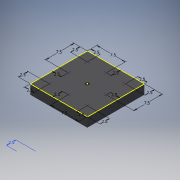
# Autodesk Inventor part: ClampCover
Saved by Autodesk Inventor 2016 (Build 200138000, 138)
## iProperties
Created: 2016-04-15
Part Number: ClampCover
Material: Generic
Document SubType Name: Modeling
Designer: Andres
Density: 1 g/cm^3
Appearance: Gray
Author: Andres
Autodesk Inventor part; units mm, degrees
ref_plane "YZ Plane" through (0, 0, 0) normal (1, 0, 0) x (0, 1, 0)
ref_plane "XZ Plane" through (0, 0, 0) normal (0, 1, 0) x (-1, 0, 0)
ref_plane "XY Plane" through (0, 0, 0) normal (0, 0, 1) x (1, 0, 0)
sketch "Sketch1" plane through (0, 0, 0) normal (0, 0, 1) x (1, 0, 0)
  line L0 (-7.5, 7.5) -> (7.5, 7.5)
  line L1 (7.5, 7.5) -> (7.5, -7.5)
  line L2 (7.5, -7.5) -> (-7.5, -7.5)
  line L3 (-7.5, -7.5) -> (-7.5, 7.5)
  point P0 (0, 0)
  point P1 (-7.5, 0)
  point P2 (0, 7.5)
  dimension "d0" = 15
  dimension "d1" = 15
  constraints: 8 end point, 2 midpoint, 2 parallel, 1 horizontal, 1 horizontal alignment, 1 perpendicular, 1 vertical alignment
  measures "d0" distance of L0.start L0.end
  measures "d1" distance of L0.end L1.end
extrude "Extrusion1" add sketch "Sketch1" along normal blind 2.5
sketch "Sketch2" plane through (0, 0, 2.5) normal (0, 0, 1) x (1, 0, 0)
  circle A0 centre (0, 0) radius 0.5
  dimension "d4" = 0.5
  constraints: 1 centre point, 1 coincident
  measures "d4" radius of A0
extrude "Extrusion2" cut sketch "Sketch2" against normal blind 2.5
sketch "Sketch3" plane through (0, 0, 2.5) normal (0, 0, 1) x (1, 0, 0)
  line L0 (7.5, -7.5) -> (-7.5, -7.5) projected
  line L1 (7.5, -7.5) -> (7.5, 7.5) projected
  line L2 (-7.5, 7.5) -> (-7.5, -7.5) projected
  line L3 (7.5, 7.5) -> (-7.5, 7.5) projected
  point P0 (0, 0)
  point P1 (5, -5)
  point P2 (-5, -5)
  point P3 (5, 5)
  point P4 (-5, 5)
  point P5 (5, 0)
  point P6 (-5, 0)
  point P7 (0, -5)
  point P8 (0, 5)
  dimension "d7" = 2.5
  dimension "d8" = 2.5
  dimension "d9" = 2.5
  dimension "d10" = 2.5
  dimension "d11" = 2.5
  dimension "d12" = 2.5
  dimension "d13" = 2.5
  dimension "d14" = 2.5
  dimension "d15" = 2.5
  dimension "d16" = 7.5
  dimension "d17" = 2.5
  dimension "d18" = 7.5
  dimension "d19" = 2.5
  dimension "d20" = 7.5
  dimension "d21" = 2.5
  dimension "d22" = 7.5
  measures "d7" distance from line of L0 point (5, -5)
  measures "d8" distance from line of L1 point (5, -5)
  measures "d9" distance from line of L0 point (-5, -5)
  measures "d10" distance from line of L2 point (-5, -5)
  measures "d11" distance from line of L3 point (5, 5)
  measures "d12" distance from line of L1 point (5, 5)
  measures "d13" distance from line of L2 point (-5, 5)
  measures "d14" distance from line of L3 point (-5, 5)
  measures "d15" distance from line of L0 point (0, -5)
  measures "d16" distance from line of L1 point (0, -5)
  measures "d17" distance from line of L2 point (-5, 0)
  measures "d18" distance from line of L3 point (-5, 0)
  measures "d19" distance from line of L3 point (0, 5)
  measures "d20" distance from line of L2 point (0, 5)
  measures "d21" distance from line of L1 point (5, 0)
  measures "d22" distance from line of L3 point (5, 0)
sketch "Sketch5" plane through (0, 0, 2.5) normal (0, 0, 1) x (1, 0, 0)
  point P0 (-5, -5)
  point P1 (5, 5)
  point P2 (-5, 5)
  point P3 (5, 0)
  point P4 (-5, 0)
  point P5 (0, -5)
  point P6 (0, 5)
  point P7 (5, -5)
hole "Hole2" at (-5, -5, 2.5) at (5, 5, 2.5) at (-5, 5, 2.5) at (5, 0, 2.5) at (-5, 0, 2.5) at (0, -5, 2.5) at (0, 5, 2.5) at (5, -5, 2.5) direction (0, 0, -1) diameter 1.8 depth 2.5 countersink diameter 3.6 countersink angle 90
body "Solid1"
